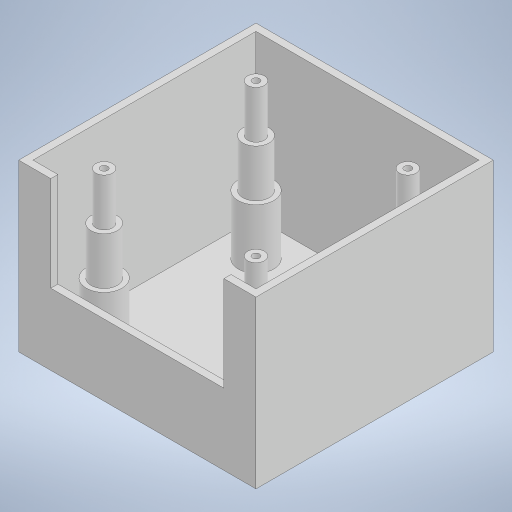
# Autodesk Inventor part: Base
Saved by Autodesk Inventor 2024.1 (Build 281209000, 209)
## iProperties
Created: 2023-12-23
Part Number: Base
Material: Generic
Document SubType Name: Modeling
Designer: ryanm
Density: 1 g/cm^3
Appearance: Default
Author: ryanm
Autodesk Inventor part; units mm, degrees
ref_plane "YZ Plane" through (0, 0, 0) normal (1, 0, 0) x (0, 1, 0)
ref_plane "XZ Plane" through (0, 0, 0) normal (0, 1, 0) x (-1, 0, 0)
ref_plane "XY Plane" through (0, 0, 0) normal (0, 0, 1) x (1, 0, 0)
sketch "Sketch1" plane through (0, 0, 0) normal (0, 1, 0) x (-1, 0, 0)
  line L0 (50, -50) -> (-50, -50)
  line L1 (-50, -50) -> (-50, 50)
  line L2 (-50, 50) -> (50, 50)
  line L3 (50, 50) -> (50, -50)
  point P0 (0, 0)
  point P1 (0, -50)
  point P2 (50, 0)
  dimension "d2" = 100
  dimension "d3" = 100
  constraints: 8 end point, 2 midpoint, 2 parallel, 1 horizontal, 1 horizontal alignment, 1 perpendicular, 1 vertical alignment
  measures "d2" distance of L0.start L0.end
  measures "d3" distance of L2.end L0.start
extrude "Extrusion1" add sketch "Sketch1" along normal blind 2
sketch "Sketch2" plane through (0, 2, 0) normal (0, 1, 0) x (1, 0, 0)
  line L0 (-50, -50) -> (50, -50) projected
  line L1 (50, -50) -> (50, 50) projected
  line L2 (50, 50) -> (-50, 50) projected
  line L3 (-50, 50) -> (-50, -50) projected
  line L4 (-47, 47) -> (47, 47)
  line L5 (47, 47) -> (47, -47)
  line L6 (47, -47) -> (-47, -47)
  line L7 (-47, -47) -> (-47, 47)
  point P0 (0, 0)
  dimension "d6" = 3
  constraints: 8 end point, 3 other
  measures "d6" distance between parallel lines of L2 L4
extrude "Extrusion2" add sketch "Sketch2" along normal blind 68
sketch "Sketch3" plane through (0, 2, 0) normal (0, 1, 0) x (1, 0, 0)
  circle A0 centre (-32, 32) radius 7.5
  circle A1 centre (32, 32) radius 7.5
  circle A2 centre (32, -32) radius 7.5
  circle A3 centre (-32, -32) radius 7.5
  line L0 (-47, 47) -> (47, 47) projected
  line L1 (-47, -47) -> (-47, 47) projected
  line L2 (47, 47) -> (47, -47) projected
  line L3 (47, -47) -> (-47, -47) projected
  point P0 (0, 0)
  dimension "d9" = 15
  dimension "d10" = 15
  dimension "d11" = 15
  dimension "d12" = 15
  dimension "d13" = 15
  dimension "d14" = 15
  dimension "d15" = 15
  dimension "d16" = 15
  constraints: 4 centre point, 2 horizontal alignment, 2 vertical alignment
  measures "d9" diameter of A0
  measures "d10" diameter of A1
  measures "d11" diameter of A2
  measures "d12" diameter of A3
  measures "d13" distance from line of L0 A0.centre
  measures "d14" distance from line of L1 A0.centre
  measures "d15" distance from line of L2 A2.centre
  measures "d16" distance from line of L3 A2.centre
extrude "Extrusion3" add sketch "Sketch3" along normal blind 25 contours A0 | A1 | A2 | A3
sketch "Sketch4" plane through (-32, 27, -32) normal (0, 1, 0) x (1, 0, 0)
  circle A0 centre (0, 0) radius 7.5 projected
  circle A1 centre (64, 0) radius 7.5 projected
  circle A2 centre (64, -64) radius 7.5 projected
  circle A3 centre (0, -64) radius 7.5 projected
  circle A4 centre (0, 0) radius 5.5
  circle A5 centre (64, 0) radius 5.5
  circle A6 centre (64, -64) radius 5.5
  circle A7 centre (0, -64) radius 5.5
  point P0 (32, -32)
  dimension "d19" = 2
  dimension "d21" = 2
  dimension "d22" = 2
  dimension "d23" = 2
  constraints: 4 centre point
  measures "d19" radial gap between concentric circles of A0 A4
  measures "d21" radial gap between concentric circles of A3 A7
  measures "d22" radial gap between concentric circles of A6 A2
  measures "d23" radial gap between concentric circles of A1 A5
extrude "Extrusion4" add sketch "Sketch4" along normal blind 20 contours A4 | A5 | A6 | A7
sketch "Sketch5" plane through (-32, 47, 32) normal (0, 1, 0) x (1, 0, 0)
  circle A0 centre (0, 64) radius 5.5 projected
  circle A1 centre (64, 64) radius 5.5 projected
  circle A2 centre (64, 0) radius 5.5 projected
  circle A3 centre (0, 0) radius 5.5 projected
  circle A4 centre (0, 64) radius 3.5
  circle A5 centre (64, 64) radius 3.5
  circle A6 centre (64, 0) radius 3.5
  circle A7 centre (0, 0) radius 3.5
  point P0 (32, 32)
  dimension "d26" = 2
  dimension "d27" = 2
  dimension "d28" = 2
  dimension "d29" = 2
  constraints: 4 centre point
  measures "d26" radial gap between concentric circles of A0 A4
  measures "d27" radial gap between concentric circles of A1 A5
  measures "d28" radial gap between concentric circles of A2 A6
  measures "d29" radial gap between concentric circles of A3 A7
extrude "Extrusion5" add sketch "Sketch5" along normal blind 20 contours A4 | A5 | A6 | A7
sketch "Sketch6" plane through (-50, 0, 50) normal (0, 0, 1) x (1, 0, 0)
  line L0 (25.5, 27) -> (10.5, 27) projected
  line L1 (89.5, 27) -> (74.5, 27) projected
  line L2 (13.5, 30) -> (86.5, 30)
  line L3 (13.5, 30) -> (13.5, 70)
  line L4 (14.5, 47) -> (14.5, 67) projected
  line L5 (13.5, 70) -> (86.5, 70)
  line L6 (86.5, 70) -> (86.5, 30)
  point P0 (50, 0)
  point P1 (0, 70)
  dimension "d32" = 3
  dimension "d33" = 3
  dimension "d34" = 3
  constraints: 8 end point, 2 perpendicular, 1 horizontal, 1 horizontal alignment, 1 parallel
  measures "d32" distance between parallel lines of L2 L0
  measures "d33" horizontal distance of L1.start L2.end
  measures "d34" horizontal distance of L2.start L0.end
extrude "Extrusion6" cut sketch "Sketch6" against normal up to surface (3 mm away)
sketch "Sketch7" plane through (-32, 67, -32) normal (0, 1, 0) x (1, 0, 0)
  circle A0 centre (0, 0) radius 3.5 projected
  circle A1 centre (0, -64) radius 3.5 projected
  circle A2 centre (64, -64) radius 3.5 projected
  circle A3 centre (64, 0) radius 3.5 projected
  point P0 (32, -32)
  constraints: 4 coincident
hole "Hole1" at (-32, 67, -32) at (32, 67, -32) at (32, 67, 32) at (-32, 67, 32) direction (0, -1, 0) diameter 3 depth 8 tip angle 118
equation "\"d10\" = d9"
equation "\"d11\" = d9"
equation "\"d12\" = d9"
equation "\"d14\" = d13"
equation "\"d15\" = d13"
equation "\"d16\" = d14"
equation "\"d21\" = d19"
equation "\"d22\" = d19"
equation "\"d23\" = d19"
body "Solid1"
